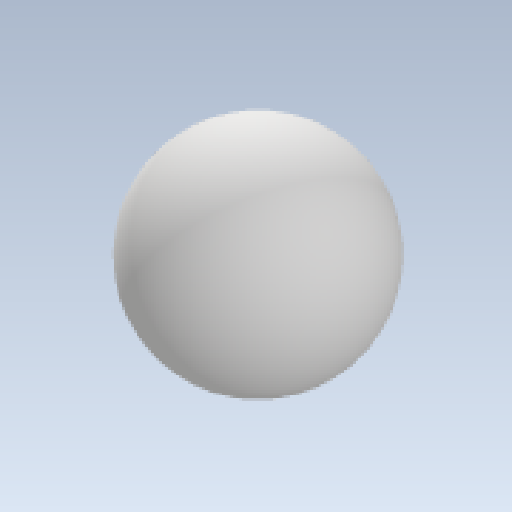
# Autodesk Inventor part: bolder
Saved by Autodesk Inventor 2023 (Build 270158030, 158C)
## iProperties
Created: 2024-12-20
Part Number: bolder
Material: Generic
Document SubType Name: Modeling
Designer: Imogen Heard
Density: 1 g/cm^3
Appearance: Default
Author: Imogen Heard
Autodesk Inventor part; units mm, degrees
ref_plane "YZ Plane" through (0, 0, 0) normal (1, 0, 0) x (0, 1, 0)
ref_plane "XZ Plane" through (0, 0, 0) normal (0, 1, 0) x (-1, 0, 0)
ref_plane "XY Plane" through (0, 0, 0) normal (0, 0, 1) x (1, 0, 0)
sketch "Sketch1" plane through (0, 0, 0) normal (1, 0, 0) x (0, 1, 0)
  circle A0 centre (0, 7) radius 12.5
  line L0 (12.5, 7) -> (-12.5, 7)
  line L1 (-12.5, 7) -> (-12.5, -5)
  line L2 (-12.5, -5) -> (12.5, -5)
  line L3 (12.5, -5) -> (12.5, 7)
  line L4 (37.5, -5) -> (17.5, -5) projected
  line L5 (0, 21.5767) -> (0, -9.94)
  point P0 (0, 0)
  point P1 (0, 19.5)
  point P2 (0, -5)
  point P3 (3.5, -5)
  dimension "d0" = 25
  dimension "d1" = 12
  constraints: 10 end point, 2 horizontal alignment, 2 parallel, 2 point on circle, 2 vertical alignment, 1 centre point, 1 horizontal, 1 midpoint, 1 perpendicular, 1 vertical
  measures "d0" diameter of A0
  measures "d1" distance between parallel lines of L2 L0
revolve "Revolution1" add sketch "Sketch1" angle 360 about axis through (0, 0, 21.5767) along (0, 0, -1) picked at (0.9272, 15.2289) picked at (1.1667, -1) contours L0 L5 A0 | A0 L2 L5 L0
body "Solid1"
